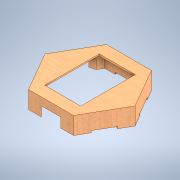
# Autodesk Inventor part: Hexagone
Saved by Autodesk Inventor 2020 (Build 240168000, 168)
## iProperties
Created: 2020-04-08
Part Number: Hexagone
Material: Wood (Cherry)
Document SubType Name: Modeling
Designer: Samuele
Density: 0.63 g/cm^3
Appearance: Cherry - Natural Low Gloss
Author: Samuele
Autodesk Inventor part; units mm, degrees
ref_plane "YZ Plane" through (0, 0, 0) normal (1, 0, 0) x (0, 1, 0)
ref_plane "XZ Plane" through (0, 0, 0) normal (0, 1, 0) x (-1, 0, 0)
ref_plane "XY Plane" through (0, 0, 0) normal (0, 0, 1) x (1, 0, 0)
sketch "Sketch6" plane through (0, 0, 0) normal (0, 1, 0) x (-1, 0, 0)
  line L0 (4.5, -6.1) -> (60.5, -6.1)
  line L1 (60.5, -6.1) -> (60.5, -90.9)
  line L2 (4.5, -90.9) -> (4.5, -6.1)
  line L3 (65.1201, -97) -> (0, -97)
  line L4 (0, -97) -> (0, 0)
  line L5 (0, 0) -> (65.1201, 0)
  line L6 (65.1201, 0) -> (65.1201, -97)
  line L7 (60.5, -90.9) -> (4.5, -90.9)
  line L8 (102.5, -48.5) -> (-37.5, -48.5)
  line L9 (32.5, -118.5) -> (32.5, 21.5)
  circle A0 centre (32.5, -48.5) radius 70
  line L10 (102.5, -48.5) -> (67.5, -109.1218)
  line L11 (67.5, -109.1218) -> (-2.5, -109.1218)
  line L12 (-2.5, -109.1218) -> (-37.5, -48.5)
  line L13 (-37.5, -48.5) -> (-2.5, 12.1218)
  line L14 (-2.5, 12.1218) -> (67.5, 12.1218)
  line L15 (67.5, 12.1218) -> (102.5, -48.5)
  line L16 (32.5, 12.1218) -> (85, -18.1891)
  line L17 (85, -18.1891) -> (85, -78.8109)
  line L18 (85, -78.8109) -> (32.5, -109.1218)
  line L19 (32.5, -109.1218) -> (-20, -78.8109)
  line L20 (-20, -78.8109) -> (-20, -18.1891)
  line L21 (-20, -18.1891) -> (32.5, 12.1218)
  line L22 (32.5, 12.1218) -> (47.5, 12.1218)
  line L23 (47.5, 12.1218) -> (47.5, 5.6218)
  line L24 (47.5, 5.6218) -> (17.5, 5.6218)
  line L25 (17.5, 5.6218) -> (17.5, 12.1218)
  line L26 (47.5, 5.6218) -> (56.6924, 5.6218) construction
  line L27 (17.5, 8.8718) -> (20, 8.8718)
  line L28 (47.5, 8.8718) -> (45, 8.8718)
  line L29 (45, 8.8718) -> (45, 10.1218)
  line L30 (45, 10.1218) -> (20, 10.1218)
  line L31 (20, 10.1218) -> (20, 7.6218)
  line L32 (20, 7.6218) -> (45, 7.6218)
  line L33 (45, 7.6218) -> (45, 10.1218)
  line L34 (67.5, 12.1218) -> (32.5, -48.5)
  line L35 (32.5, -48.5) -> (67.5, -109.1218)
  line L36 (47.5, 5.6218) -> (56.6924, 5.6218)
  line L37 (17.5, 5.6218) -> (11, 5.6218)
  line L38 (17.5, 12.1218) -> (11, 5.6218)
  line L39 (17.5, 12.1218) -> (26.6924, 12.1218) construction
  line L40 (47.5, 12.1218) -> (54, 5.6218)
  line L41 (85, -18.1891) -> (77.5, -5.1987)
  line L42 (77.5, -5.1987) -> (71.8708, -8.4487)
  line L43 (71.8708, -8.4487) -> (86.8708, -34.4295)
  line L44 (86.8708, -34.4295) -> (92.5, -31.1795)
  line L45 (71.8708, -8.4487) -> (67.2746, -0.4879) construction
  line L46 (89.6854, -32.8045) -> (88.4354, -30.6394)
  line L47 (74.6854, -6.8237) -> (75.9354, -8.9888)
  line L48 (75.9354, -8.9888) -> (77.0179, -8.3638)
  line L49 (77.0179, -8.3638) -> (89.5179, -30.0144)
  line L50 (89.5179, -30.0144) -> (87.3529, -31.2644)
  line L51 (87.3529, -31.2644) -> (74.8529, -9.6138)
  line L52 (74.8529, -9.6138) -> (77.0179, -8.3638)
  line L53 (71.8708, -8.4487) -> (67.2746, -0.4879)
  line L54 (86.8708, -34.4295) -> (90.1208, -40.0587)
  line L55 (92.5, -31.1795) -> (90.1208, -40.0587)
  line L56 (92.5, -31.1795) -> (87.9038, -23.2187) construction
  line L57 (77.5, -5.1987) -> (68.6208, -2.8196)
  line L58 (71.8708, -88.5513) -> (67.2746, -96.5121) construction
  line L59 (74.6854, -90.1763) -> (75.9354, -88.0112)
  line L60 (74.8529, -87.3862) -> (77.0179, -88.6362)
  line L61 (77.5, -91.8013) -> (71.8708, -88.5513)
  line L62 (77.5, -91.8013) -> (68.6208, -94.1804)
  line L63 (71.8708, -88.5513) -> (67.2746, -96.5121)
  line L64 (77.0179, -88.6362) -> (89.5179, -66.9856)
  line L65 (87.3529, -65.7356) -> (74.8529, -87.3862)
  line L66 (71.8708, -88.5513) -> (86.8708, -62.5705)
  line L67 (89.5179, -66.9856) -> (87.3529, -65.7356)
  line L68 (89.6854, -64.1955) -> (88.4354, -66.3606)
  line L69 (86.8708, -62.5705) -> (92.5, -65.8205)
  line L70 (86.8708, -62.5705) -> (90.1208, -56.9413)
  line L71 (92.5, -65.8205) -> (90.1208, -56.9413)
  line L72 (94.9944, -48.5) -> (63.7472, -102.6218)
  line L73 (63.7472, -102.6218) -> (1.2528, -102.6218)
  line L74 (1.2528, -102.6218) -> (-29.9944, -48.5)
  line L75 (-29.9944, -48.5) -> (1.2528, 5.6218)
  line L76 (1.2528, 5.6218) -> (63.7472, 5.6218)
  line L77 (63.7472, 5.6218) -> (94.9944, -48.5)
  line L78 (74.8529, -87.3862) -> (73.1208, -86.3862)
  line L79 (87.3529, -65.7356) -> (85.6208, -64.7356)
  line L80 (87.3529, -31.2644) -> (85.6208, -32.2644)
  line L81 (74.8529, -9.6138) -> (73.1208, -10.6138)
  line L82 (45, 7.6218) -> (45, 5.6218)
  line L83 (20, 7.6218) -> (20, 5.6218)
  line L84 (60.5, -90.9) -> (4.4985, -90.9)
  line L85 (4.4985, -90.9) -> (4.4985, -97)
  line L86 (4.4985, -97) -> (60.5, -97)
  line L87 (60.5, -97) -> (60.5, -90.9)
  line L88 (60.5, -6.1) -> (4.4985, -6.1)
  line L89 (4.4985, -6.1) -> (4.4985, 0)
  line L90 (4.4985, 0) -> (60.5, 0)
  line L91 (60.5, 0) -> (60.5, -6.1)
  dimension "d44" = 97
  dimension "d77" = 140
  dimension "d87" = 15
  dimension "d88" = 6.5
  dimension "d89" = 30
  dimension "d91" = 2.5
  dimension "d92" = 2.5
  dimension "d95" = 1.25
  dimension "d96" = 25
  dimension "d97" = 2.5
  dimension "d98" = 25
  dimension "d99" = 135
  dimension "d100" = 0
  constraints: 184 end point, 37 symmetric about line, 15 point on line, 12 horizontal, 12 perpendicular, 9 parallel, 5 midpoint, 5 vertical, 4 point on circle, 3 coincident, 2 collinear, 1 centre point, 1 equal length, 1 horizontal alignment, 42 other
  measures "d44" distance of L5.end L3.start
  measures "d77" diameter of A0
  measures "d87" distance of L16.start L22.end
  measures "d88" distance of L22.end L23.end
  measures "d89" distance of L23.end L24.end
  measures "d91" distance of L27.start L27.end
  measures "d92" distance of L28.start L28.end
  measures "d95" distance of L28.end L29.end
  measures "d96" distance of L29.end L30.end
  measures "d97" distance of L30.end L31.end
  measures "d98" distance of L31.end L32.end
  measures "d99" angle of L38 L39
  measures "d100" distance of L25.end L38.start
extrude "Fronte" add sketch "Sketch6" along normal blind 2 contours L89 L21 L5 L9 L0 | L2 L8 L4 L21 L89 | L9 L5 L16 L34 L0 | L2 L85 L19 L4 L8 | L89 L5 L21 | L21 L4 L5 L89 | L34 L16 L91 L0 | L9 L24 L16 L5 | L5 L21 L24 L9 | L7 L9 L3 L19 L85 | L8 L20 L75 L21 L4 | L4 L19 L74 L20 L8 | L21 L75 L76 L37 L24 L5 L4 | L91 L16 L6 L8 L1 | L34 L91 L16 | L16 L5 L34 | L8 L6 L18 L87 L1 | L7 L35 L18 L3 L9 | L7 L87 L18 L35 | L16 L24 L36 L76 L34 L5 | L24 L21 L32 L9 | L9 L32 L16 L24 | L85 L3 L4 L19 | L19 L3 L85 | L4 L3 L19 L73 L74 | L20 L74 L8 | L8 L75 L20 | L75 L20 L21 | L21 L13 L14 L38 L76 L75 | L24 L83 L32 L21 | L91 L5 L6 L16 | L34 L77 L53 L43 L16 L6 L5 | L8 L17 L66 L18 L6 | L6 L16 L43 L17 L8 | L9 L73 L19 L3 | L3 L18 L73 L9 | L35 L3 L18 | L18 L87 L35 | L16 L32 L82 L24 | L32 L21 L30 L9 | L9 L30 L16 L32 | L74 L73 L19 L11 L12 | L19 L20 L74 | L74 L20 L12 L8 | L8 L13 L20 L75 | L32 L31 L30 L21 | L24 L25 L27 L31 L83 | L76 L36 L40 L14 L34 | L34 L15 L57 L53 L77 | L18 L6 L3 L87 | L18 L66 L63 L72 L35 L3 L6 | L17 L43 L54 L77 L8 | L8 L72 L70 L66 L17 | L3 L35 L73 L18 | L73 L18 L9 | L9 L19 L73 | L16 L30 L29 L33 L32 | L82 L33 L28 L23 L24 | L30 L21 L9 | L9 L16 L30 | L38 L25 L37 | L30 L31 L27 L25 L14 L21 | L43 L81 L51 L16 | L16 L51 L17 L43 | L66 L17 L65 L18 | L18 L65 L78 L66 | L77 L55 L15 L8 | L8 L10 L71 L72 | L17 L51 L80 L43 | L66 L79 L65 L17 | L73 L35 L11 L18 | L72 L63 L62 L10 L35 | L16 L14 L23 L28 L29 L30 | L23 L40 L36 | L51 L52 L48 L49 L16 | L16 L49 L17 L51 | L43 L42 L47 L52 L81 | L15 L16 L49 L48 L47 L42 | L42 L53 L57 | L65 L17 L64 L18 | L18 L64 L60 L65 | L78 L60 L59 L61 L66 | L71 L69 L70 | L54 L44 L55 | L17 L49 L50 L51 | L80 L50 L46 L44 L43 | L65 L67 L64 L17 | L66 L69 L68 L67 L79 | L16 L17 L49 | L10 L17 L64 L67 L68 L69 | L44 L46 L50 L49 L17 L15 | L64 L17 L18 | L18 L10 L61 L59 L60 L64 | L61 L62 L63
extrude "Esterno" add sketch "Sketch6" against normal blind 25 contours L75 L20 L21 | L21 L13 L14 L38 L76 L75 | L74 L73 L19 L11 L12 | L19 L20 L74 | L74 L20 L12 L8 | L8 L13 L20 L75 | L76 L36 L40 L14 L34 | L34 L15 L57 L53 L77 | L73 L18 L9 | L9 L19 L73 | L77 L55 L15 L8 | L8 L10 L71 L72 | L73 L35 L11 L18 | L72 L63 L62 L10 L35
extrude "Strip" add sketch "Sketch6" against normal blind 10 contours L24 L21 L32 L9 | L9 L32 L16 L24 | L24 L83 L32 L21 | L16 L32 L82 L24 | L24 L25 L27 L31 L83 | L82 L33 L28 L23 L24 | L30 L21 L9 | L9 L16 L30 | L38 L25 L37 | L30 L31 L27 L25 L14 L21 | L43 L81 L51 L16 | L16 L51 L17 L43 | L66 L17 L65 L18 | L18 L65 L78 L66 | L17 L51 L80 L43 | L66 L79 L65 L17 | L16 L14 L23 L28 L29 L30 | L23 L40 L36 | L43 L42 L47 L52 L81 | L15 L16 L49 L48 L47 L42 | L42 L53 L57 | L78 L60 L59 L61 L66 | L71 L69 L70 | L54 L44 L55 | L80 L50 L46 L44 L43 | L66 L69 L68 L67 L79 | L16 L17 L49 | L10 L17 L64 L67 L68 L69 | L44 L46 L50 L49 L17 L15 | L64 L17 L18 | L18 L10 L61 L59 L60 L64 | L61 L62 L63
sketch "Sketch7" plane through (0, -25, 0) normal (0, -1, 0) x (1, 0, 0)
  line L0 (-17.5, 12.1218) -> (-17.5, -109.1218)
  line L1 (-67.5, -109.1218) -> (2.5, -109.1218) projected
  line L2 (-47.5, 12.1218) -> (-67.5, 12.1218) projected
  line L3 (-47.5, 12.1218) -> (-47.5, -109.1218)
  line L4 (-77.5, -91.8013) -> (-67.5, -109.1218) projected
  line L5 (-77.5, -91.8013) -> (27.5, -31.1795)
  line L6 (2.5, 12.1218) -> (37.5, -48.5) projected
  line L7 (-92.5, -65.8205) -> (-90.1208, -56.9413) projected
  line L8 (-92.5, -65.8205) -> (12.5, -5.1987)
  line L9 (-77.5, -5.1987) -> (27.5, -65.8205)
  line L10 (37.5, -48.5) -> (2.5, -109.1218) projected
  line L11 (-92.5, -31.1795) -> (11.423, -93.6666)
  line L12 (27.5, -31.1795) -> (12.5, -5.1987)
  line L13 (27.5, -65.8205) -> (11.423, -93.6666)
  line L14 (-1.2528, -102.6218) -> (29.9944, -48.5) projected
  line L15 (5.8516, -90.3166) -> (21.8708, -62.5705)
  line L16 (-47.5, -109.1218) -> (-17.5, -109.1218)
  line L17 (-17.5, -109.1218) -> (-17.5, -102.6218)
  line L18 (-17.5, -102.6218) -> (-47.5, -102.6218)
  line L19 (-47.5, -102.6218) -> (-47.5, -109.1218)
  line L20 (5.5339, -9.2206) -> (17.5, -36.953)
  point P0 (0, 0)
  point P1 (6.9325, -8.4131)
  point P2 (21.9325, -34.3939)
  constraints: 28 end point, 13 point on line, 3 parallel, 2 vertical, 1 horizontal, 1 perpendicular
extrude "Passacavi" cut sketch "Sketch7" against normal blind 3 contours L0 L1 L3 L18 | L14 L9 L10 L11 | L20 L8 L6 L5
extrude "ScavoStrip" cut sketch "Sketch6" against normal blind 5 contours L24 L21 L32 L9 | L9 L32 L16 L24 | L24 L83 L32 L21 | L16 L32 L82 L24 | L43 L81 L51 L16 | L16 L51 L17 L43 | L66 L17 L65 L18 | L18 L65 L78 L66 | L17 L51 L80 L43 | L66 L79 L65 L17
extrude "ScreenDis1" add sketch "Sketch6" against normal blind 1 contours L7 L9 L3 L19 L85 | L7 L35 L18 L3 L9 | L7 L87 L18 L35 | L19 L3 L85 | L35 L3 L18 | L18 L87 L35
extrude "ScreenDist1.8" add sketch "Sketch6" against normal blind 1.8 contours L89 L21 L5 L9 L0 | L9 L5 L16 L34 L0 | L89 L5 L21 | L34 L16 L91 L0 | L34 L91 L16 | L16 L5 L34
body "Solid3"
